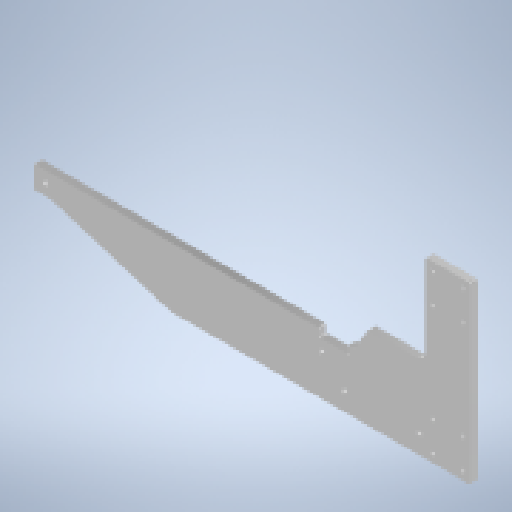
# Autodesk Inventor part: Z-Axis Support Plates
Saved by Autodesk Inventor 2024 (Build 280153000, 153)
## iProperties
Created: 2024-12-30
Part Number: Z-Axis Support Plates
Material: Aluminum 6061
Document SubType Name: Modeling
Designer: Ishaan
Density: 2.7 g/cm^3
Appearance: Aluminum - Flat
Author: Ishaan
Autodesk Inventor part; units mm, degrees
ref_plane "YZ Plane" through (0, 0, 0) normal (1, 0, 0) x (0, 1, 0)
ref_plane "XZ Plane" through (0, 0, 0) normal (0, 1, 0) x (-1, 0, 0)
ref_plane "XY Plane" through (0, 0, 0) normal (0, 0, 1) x (1, 0, 0)
sketch "Sketch1" plane through (0, 0, 0) normal (0, 0, 1) x (1, 0, 0)
  line L0 (191.375, -26.35) -> (-191.375, -26.35)
  line L1 (-191.375, -26.35) -> (-191.375, 26.35)
  line L2 (-191.375, 26.35) -> (191.375, 26.35)
  line L3 (191.375, 26.35) -> (191.375, -26.35)
  line L4 (191.375, -26.35) -> (-191.375, 26.35) construction
  line L5 (-191.375, -26.35) -> (191.375, 26.35) construction
  line L6 (-191.375, 26.35) -> (-171.375, 26.35)
  line L7 (-171.375, 26.35) -> (-171.375, 6.35)
  line L8 (-171.375, 6.35) -> (-191.375, 6.35)
  line L9 (-191.375, 6.35) -> (-191.375, 26.35)
  line L10 (-176.375, 6.35) -> (-71.375, -26.35)
  line L11 (-181.375, 6.35) -> (-181.375, 46.2875) construction
  line L12 (71.125, 20) -> (91.125, 20)
  line L13 (91.125, 20) -> (91.125, -20)
  line L14 (91.125, -20) -> (71.125, -20)
  line L15 (71.125, -20) -> (71.125, 20)
  line L16 (-190.125, 46.2875) -> (79.875, 46.2875) construction
  line L17 (79.875, 46.2875) -> (79.875, 38.35) construction
  line L18 (79.875, 38.35) -> (-190.125, 38.35) construction
  line L19 (-190.125, 38.35) -> (-190.125, 46.2875) construction
  line L20 (71.125, 46.2875) -> (-181.375, 46.2875) construction
  line L21 (191.375, -26.35) -> (151.375, -26.35)
  line L22 (151.375, -26.35) -> (151.375, 13.65)
  line L23 (151.375, 13.65) -> (191.375, 13.65)
  line L24 (191.375, 13.65) -> (191.375, -26.35)
  line L25 (191.375, -26.35) -> (151.375, 13.65) construction
  line L26 (151.375, -26.35) -> (191.375, 13.65) construction
  line L27 (184.375, -19.35) -> (158.375, -19.35) construction
  line L28 (158.375, -19.35) -> (158.375, 6.65) construction
  line L29 (158.375, 6.65) -> (184.375, 6.65) construction
  line L30 (184.375, 6.65) -> (184.375, -19.35) construction
  line L31 (184.375, -19.35) -> (158.375, 6.65) construction
  line L32 (158.375, -19.35) -> (184.375, 6.65) construction
  line L33 (191.375, 86.65) -> (151.375, 86.65)
  line L34 (151.375, 86.65) -> (151.375, 126.65)
  line L35 (151.375, 126.65) -> (191.375, 126.65)
  line L36 (191.375, 126.65) -> (191.375, 86.65)
  line L37 (191.375, 86.65) -> (151.375, 126.65) construction
  line L38 (151.375, 86.65) -> (191.375, 126.65) construction
  line L39 (184.375, 93.65) -> (158.375, 93.65) construction
  line L40 (158.375, 93.65) -> (158.375, 119.65) construction
  line L41 (158.375, 119.65) -> (184.375, 119.65) construction
  line L42 (184.375, 119.65) -> (184.375, 93.65) construction
  line L43 (184.375, 93.65) -> (158.375, 119.65) construction
  line L44 (158.375, 93.65) -> (184.375, 119.65) construction
  line L45 (191.375, 86.65) -> (191.375, 26.35)
  line L46 (151.375, 86.65) -> (151.375, 13.65)
  line L47 (171.375, -6.35) -> (211.375, -6.35) construction
  line L48 (-181.375, 26.3188) -> (-181.375, 6.35) construction
  line L49 (156.125, -20) -> (136.125, -20)
  line L50 (136.125, -20) -> (136.125, 0)
  line L51 (136.125, 0) -> (156.125, 0)
  line L52 (156.125, 0) -> (156.125, -20)
  line L53 (156.125, -20) -> (136.125, 0) construction
  line L54 (136.125, -20) -> (156.125, 0) construction
  line L55 (91.125, 20) -> (51.125, 20)
  line L56 (51.125, 20) -> (51.125, 0)
  line L57 (51.125, 0) -> (91.125, 0)
  line L58 (91.125, 0) -> (91.125, 20)
  line L59 (151.375, 46.35) -> (101.375, 46.35)
  line L60 (101.375, 46.35) -> (89.828, 26.35)
  point P0 (0, 0)
  point P1 (71.125, 0)
  point P2 (-55.125, 46.2875)
  point P3 (171.375, 106.65)
  point P4 (116.734, 26.35)
  point P5 (61.125, 10)
  point P6 (81.125, -10)
  point P7 (91.125, 0)
  point P8 (88.5805, 0)
  point P9 (81.125, 20)
  point P10 (146.125, -10)
  point P11 (146.125, -10)
  point P12 (51.125, 10)
  point P13 (81.125, -20)
  point P14 (-181.375, 16.35)
  point P15 (-191.375, 16.35)
  point P16 (-171.375, 26.35)
  point P17 (151.375, 26.35)
  dimension "d0" = 52.7
  dimension "d1" = 20
  dimension "d2" = 20
  dimension "d4" = 120
  dimension "d5" = 20
  dimension "d6" = 40
  dimension "d8" = 270
  dimension "d9" = 7.9375
  dimension "d10" = 12
  dimension "d11" = 40
  dimension "d12" = 40
  dimension "d13" = 26
  dimension "d14" = 26
  dimension "d15" = 40
  dimension "d16" = 40
  dimension "d17" = 26
  dimension "d18" = 26
  dimension "d19" = 153
  dimension "d20" = 40
  dimension "d21" = 226.5
  dimension "d22" = 15
  dimension "d35" = 20
  dimension "d47" = 20
  dimension "d48" = 20
  dimension "d49" = 45
  dimension "d57" = 252.5
  dimension "d58" = 10
  dimension "d59" = 10
  dimension "d69" = 120
  dimension "d70" = 50
  constraints: 122 end point, 22 midpoint, 20 parallel, 13 horizontal, 12 perpendicular, 9 coincident, 7 point on line, 4 horizontal alignment, 3 collinear, 1 vertical, 1 vertical alignment
  measures "d0" distance between parallel lines of L2 L0
  measures "d1" distance of L7.end L8.end
  measures "d2" distance of L6.end L7.end
  measures "d4" distance from line of L10.end L1
  measures "d5" distance of L13.end L14.end
  measures "d6" distance of L12.end L13.end
  measures "d8" distance of L17.end L18.end
  measures "d9" distance of L16.end L17.end
  measures "d10" distance between parallel lines of L18 L2
  measures "d11" distance of L22.end L23.end
  measures "d12" distance of L21.end L22.end
  measures "d13" distance of L28.end L29.end
  measures "d14" distance of L27.end L28.end
  measures "d15" distance of L34.end L35.end
  measures "d16" distance of L33.end L34.end
  measures "d17" distance of L40.end L41.end
  measures "d18" distance of L39.end L40.end
  measures "d19" distance between parallel lines of L0 L35
  measures "d20" distance of L47.start L47.end
  measures "d21" horizontal distance of point (-55.125, 46.288) L47.start
  measures "d22" distance from line of L10.start L1
  measures "d35" distance from line of L2 L59.start
  measures "d47" distance of L50.end L51.end
  measures "d48" distance of L49.end L50.end
  measures "d49" distance between parallel lines of L13 L50
  measures "d57" distance of L20.start L11.end
  measures "d58" distance from line of L14 point (81.125, -10)
  measures "d59" distance from line of L56 point (61.125, 10)
  measures "d69" angle of L59 L60
  measures "d70" distance of L59.start L59.end
extrude "Extrusion1" add sketch "Sketch1" along normal blind 6.35 contours L0 L22 L49 L52 L51 L23 L3 | L0 L10 L8 L7 L2 L46 L22 L51 L50 L49 | L23 L46 L2 L3 | L49 L50 L51 L22 | L22 L51 L52 L49 | L2 L46 L33 L45 | L8 L1 L2 L7 | L2 L60 L59 L46 | L33 L34 L35 L36 | L12 L13 L57 L15 | L15 L57 L56 L55 | L57 L13 L14 L15
fillet "Fillet2" radius 1 2 edges at (-191.375, 26.35, 3.175) (-191.375, 6.35, 3.175)
fillet "Fillet5" radius 8 1 edges at (151.375, 46.35, 3.175)
fillet "Fillet3" radius 2 7 edges at (151.375, 126.65, 3.175) (191.375, 126.65, 3.175) (191.375, -26.35, 3.175) (89.828, 26.35, 3.175) (101.375, 46.35, 3.175) (-71.375, -26.35, 3.175) (-176.375, 6.35, 3.175)
hole "Hole1" at (61.125, 10, 0) at (81.125, -10, 0) at (146.125, -10, 0) at (-181.375, 16.35, 0) direction (0, 0, 1) diameter 5.3 end through all
hole "Hole2" at (184.375, 6.65, 0) at (158.375, 6.65, 0) at (158.375, -19.35, 0) at (184.375, -19.35, 0) at (184.375, 119.65, 0) at (158.375, 119.65, 0) at (158.375, 93.65, 0) at (184.375, 93.65, 0) direction (0, 0, 1) diameter 4.3 end through all
sketch "Sketch2" plane through (0, 0, 6.35) normal (0, 0, 1) x (1, 0, 0)
  line L0 (83.875, 19.5) -> (58.375, 19.5)
  line L1 (58.375, 19.5) -> (58.375, 26.35)
  line L2 (58.375, 26.35) -> (83.875, 26.35)
  line L3 (83.875, 26.35) -> (83.875, 19.5)
  line L4 (83.875, 19.5) -> (58.375, 26.35) construction
  line L5 (58.375, 19.5) -> (83.875, 26.35) construction
  circle A0 centre (61.125, 10) radius 2.65 projected
  circle A1 centre (81.125, -10) radius 2.65 projected
  line L6 (61.125, 10) -> (81.125, -10) construction
  line L7 (88.6733, 26.35) -> (-190.375, 26.35) construction
  circle A2 centre (58.775, 19.9) radius 0.9
  circle A3 centre (83.475, 19.9) radius 0.9
  line L8 (83.475, 25.95) -> (58.775, 25.95) construction
  line L9 (58.775, 25.95) -> (58.775, 19.9) construction
  line L10 (58.775, 19.9) -> (83.475, 19.9) construction
  line L11 (83.475, 19.9) -> (83.475, 25.95) construction
  line L12 (83.475, 25.95) -> (58.775, 19.9) construction
  line L13 (58.775, 25.95) -> (83.475, 19.9) construction
  point P0 (0, 0)
  point P1 (71.125, 22.925)
  point P2 (71.125, 0)
  point P3 (119.4481, 26.35)
  point P4 (58.375, 20.7062)
  point P5 (59.5812, 19.5)
  point P6 (82.6688, 19.5)
  point P7 (83.875, 20.7062)
  point P8 (194.625, 26.35)
  point P9 (154.625, 26.35)
  point P10 (93.078, 26.35)
  dimension "d60" = 25.5
  dimension "d61" = 6.85
  dimension "d62" = 1.8
  dimension "d63" = 0.4
  dimension "d64" = 0.4
  constraints: 26 end point, 5 midpoint, 4 parallel, 2 centre point, 2 horizontal, 2 perpendicular, 1 coincident, 1 collinear, 1 equal radius, 1 horizontal alignment, 1 vertical alignment
  measures "d60" distance of L1.end L2.end
  measures "d61" distance of L0.end L1.end
  measures "d62" diameter of A2
  measures "d63" distance between parallel lines of L3 L11
  measures "d64" distance between parallel lines of L0 L10
extrude "Extrusion2" cut sketch "Sketch2" against normal through all contours L3 A3 L0 | L0 A3 L3 | L0 A2 L1 L2 L3 A3 | A2 L1 L0 | L0 L1 A2
fillet "Fillet4" radius 1 6 edges at (83.875, 20.7062, 3.175) (82.6688, 19.5, 3.175) (59.5812, 19.5, 3.175) (58.375, 20.7062, 3.175) (58.375, 26.35, 3.175) (83.875, 26.35, 3.175)
body "Solid1"
